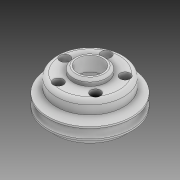
# Autodesk Inventor part: CamPlate
Saved by Autodesk Inventor 2020 (Build 240168000, 168)
## iProperties
Created: 2021-01-03
Part Number: CamPlate
Material: Generic
Document SubType Name: Modeling
Designer: DDeGo
Density: 1 g/cm^3
Appearance: Default
Author: DDeGo
Autodesk Inventor part; units mm, degrees
ref_plane "YZ Plane" through (0, 0, 0) normal (1, 0, 0) x (0, 1, 0)
ref_plane "XZ Plane" through (0, 0, 0) normal (0, 1, 0) x (-1, 0, 0)
ref_plane "XY Plane" through (0, 0, 0) normal (0, 0, 1) x (1, 0, 0)
sketch "Sketch1" plane through (0, 0, 0) normal (1, 0, 0) x (0, 1, 0)
  line L0 (0, 0) -> (8.6351, 0) construction
  line L1 (8.6351, 0) -> (8.6351, -3) construction
  line L2 (8.6351, -3) -> (6.6351, -3)
  line L3 (6.6351, -3) -> (6.6351, -1.5)
  line L4 (6.6351, -1.5) -> (4.6351, -1.5)
  line L5 (0, -1.5) -> (0, -2.6) construction
  line L6 (0, -8) -> (8.6351, -8)
  line L7 (8.6351, -8) -> (8.6351, -4)
  line L8 (0, 0) -> (0, -1.5) construction
  line L9 (8.6351, -3) -> (10.1351, -3)
  line L10 (10.1351, -3) -> (10.1351, -4)
  line L11 (10.1351, -4) -> (8.6351, -4)
  line L12 (8.6351, -4) -> (8.6351, -3) construction
  line L13 (4.6351, -1.5) -> (4.6351, -2.6) construction
  line L14 (4.6351, -2.6) -> (4, -2.6) construction
  line L15 (0, -2.6) -> (0, -8)
  line L16 (4.6351, -1.5) -> (0, -1.5) construction
  line L17 (4.6351, -1.5) -> (4, -2.6)
  line L18 (4, -2.6) -> (0, -2.6)
  dimension "d0" = 1.5
  dimension "d1" = 3
  dimension "d4" = 8
  dimension "d14" = 1
  dimension "d15" = 1.5
  dimension "d20" = 2.6
  dimension "d22" = 2
  dimension "d23" = 30
  dimension "d24" = 4
  dimension "d25" = 3.5
  dimension "d26" = 6.6351
  constraints: 38 end point, 20 perpendicular, 2 horizontal, 2 vertical, 1 point on line
  measures "d0" distance between parallel lines of L0 L4
  measures "d1" distance between parallel lines of L0 L2
  measures "d4" distance between parallel lines of L0 L6
  measures "d14" distance of L9.end L10.end
  measures "d15" distance of L10.end L7.end
  measures "d20" distance between parallel lines of L0 L14
  measures "d22" distance between parallel lines of L3 L13
  measures "d23" angle of L13 L17
  measures "d24" distance of L14.end L5.end
  measures "d25" distance between parallel lines of L3 L10
  measures "d26" distance between parallel lines of L15 L3
revolve "Revolution1" add sketch "Sketch1" angle 360 about axis through (0, 0, 0) along (0, 1, 0)
sketch "Sketch2" plane through (0, 8.6351, 0) normal (0, 1, 0) x (1, 0, 0)
  circle A0 centre (0, 0) radius 6 construction
  circle A1 centre (-6, 0) radius 1.2
  circle A2 centre (-1.8541, -5.7063) radius 1.2
  circle A3 centre (4.8541, -3.5267) radius 1.2
  circle A4 centre (4.8541, 3.5267) radius 1.2
  circle A5 centre (-1.8541, 5.7063) radius 1.2
  dimension "d6" = 12
  dimension "d7" = 2.4
  dimension "d10" = 360
  constraints: 5 centre point, 2 horizontal alignment, 1 coincident, 13 other
  measures "d7" diameter of A1
extrude "Extrusion1" cut sketch "Sketch2" against normal through all
fillet "Fillet1" radius 1 1 edges at (0, 8.6351, 8)
chamfer "Chamfer1" distance 0.6 angle 45 3 edges at (0, 10.1351, 4) (0, 0, 2.6) (0, 0, 8)
sketch "Sketch3" plane through (0, 0, 0) normal (0, 0, 1) x (1, 0, 0)
  line L0 (0, 0) -> (0, 10.1351) construction
  line L1 (-3.4, 10.1351) -> (3.4, 10.1351) construction
  line L2 (-8, 7.6351) -> (-8, 0.6) projected
  line L3 (-10, 4.5547) -> (-8, 5.5547)
  line L4 (-8, 5.5547) -> (-8, 0.6)
  line L5 (7.4, 0) -> (-7.4, 0) projected
  arc A0 (-10, 2) -> (-9.5, 3.866) centre (-10, 3) ccw
  line L6 (-10, 1.6) -> (-10, 2)
  line L7 (-10, 4) -> (-10, 4.1547) construction
  line L8 (-10, 1.6) -> (-8.4, 0)
  line L9 (-8.4, 0) -> (-7.4, 0)
  line L10 (-7.4, 0) -> (-8, 0.6)
  line L11 (-8, 0.6) -> (-7.4, 0) projected
  line L12 (-10, 4.1547) -> (-9.5, 3.866)
  arc A1 (-9.5, 3.866) -> (-10, 4) centre (-10, 3) ccw construction
  line L13 (-10, 4.1547) -> (-10, 4.5547)
  dimension "d29" = 1
  dimension "d30" = 10
  dimension "d32" = 3
  dimension "d34" = 1
  dimension "d35" = 45
  dimension "d36" = 60
  dimension "d37" = 0.4
  constraints: 20 end point, 4 collinear, 4 point on circle, 3 parallel, 2 centre point, 2 tangent, 1 horizontal, 1 midpoint, 1 point on line
  measures "d29" radius of A0
  measures "d30" distance between parallel lines of L0 L7
  measures "d32" distance from line of L5 A0.centre
  measures "d34" vertical distance of L3.start L3.end
  measures "d35" angle of L9 L8
  measures "d36" angle of L7 L12
  measures "d37" distance of L7.end L3.start
revolve "Revolution2" add sketch "Sketch3" angle 360 about axis through (0, 0, 0) along (0, 1, 0)
body "Solid1"
